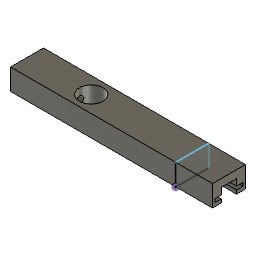
ペン抑え (Autodesk Fusion 360 design; units mm, degrees)
Autodesk Fusion 360 part; units mm, degrees
note: some values were not read from the file. Set by a fixed rule: which sketch regions a step uses.
sketch "スケッチ3" plane through (0, 0, 0) normal (0, 0, 1) x (1, 0, 0)
  line L0 (0, 0) -> (45, 0)
  line L1 (45, 0) -> (45, 9)
  line L2 (45, 9) -> (0, 9)
  line L3 (0, 9) -> (0, 0)
  dimension "d4" = 45
  dimension "d5" = 9
  constraint horizontal L0
  constraint vertical L1
  constraint horizontal L2
  constraint vertical L3
  constraint coincident L0.start L3.end
  measures "d4" distance of L0.start L0.end
  measures "d5" distance of L0.start L2.end
extrude "押し出し2" add sketch "スケッチ3" along normal blind 5.8
sketch "スケッチ4" plane through (0, 0, 0) normal (1, 0, 0) x (0, 1, 0)
sketch "スケッチ5" plane through (45, 0, 0) normal (1, 0, 0) x (0, 1, 0)
  line L0 (0, 0) -> (9, 0)
  line L1 (9, 0) -> (9, 5.8)
  line L2 (9, 5.8) -> (0, 5.8)
  line L3 (0, 5.8) -> (0, 0)
  line L4 (0, 0) -> (0.85, 0)
  line L5 (0.85, 0) -> (0.85, 5.8)
  line L6 (0.85, 5.8) -> (0, 5.8)
  line L7 (0, 5.8) -> (0, 0)
  line L8 (9, 0) -> (8.15, 0)
  line L9 (8.15, 0) -> (8.15, 5.7622)
  line L10 (8.15, 5.7622) -> (9, 5.7622)
  line L11 (9, 5.7622) -> (9, 0)
  line L12 (0.85, 0) -> (8.15, 0)
  line L13 (8.15, 0) -> (8.15, 1)
  line L14 (8.15, 1) -> (0.85, 1)
  line L15 (0.85, 1) -> (0.85, 0)
  line L16 (0.85, 5.8) -> (8.1927, 5.8)
  line L17 (8.1927, 5.8) -> (8.1927, 1.8)
  line L18 (8.1927, 1.8) -> (0.85, 1.8)
  line L19 (0.85, 1.8) -> (0.85, 5.8)
  line L20 (4.5, 1) -> (6.55, 1)
  line L21 (6.55, 1) -> (6.55, 0)
  line L22 (6.55, 0) -> (4.5, 0)
  line L23 (4.5, 0) -> (4.5, 1)
  line L24 (4.5, 0) -> (2.45, 0)
  line L25 (2.45, 0) -> (2.45, 1)
  line L26 (2.45, 1) -> (4.5, 1)
  line L27 (4.5, 1) -> (4.5, 0)
  dimension "d8" = 0.85
  dimension "d9" = 0.85
  dimension "d10" = 1
  dimension "d11" = 4
  dimension "d12" = 2.05
  dimension "d13" = 2.05
  constraint horizontal L4
  constraint vertical L5
  constraint horizontal L6
  constraint vertical L7
  constraint coincident L0.start L3.end
  constraint horizontal L8
  constraint vertical L9
  constraint horizontal L10
  constraint vertical L11
  constraint coincident L0.end L1.start
  constraint horizontal L12
  constraint vertical L13
  constraint horizontal L14
  constraint vertical L15
  constraint horizontal L16
  constraint vertical L17
  constraint horizontal L18
  constraint vertical L19
  constraint horizontal L20
  constraint vertical L21
  constraint horizontal L22
  constraint vertical L23
  constraint midpoint L14 L20.start
  constraint horizontal L24
  constraint vertical L25
  constraint horizontal L26
  constraint vertical L27
  measures "d8" distance of L0.start L4.end
  measures "d9" distance of L0.end L8.end
  measures "d10" distance of L4.end L14.end
  measures "d11" distance of L5.end L18.end
  measures "d12" distance of L20.start L20.end
  measures "d13" distance of L22.end L24.end
sketch "スケッチ6" plane through (0, 0, 5.8) normal (0, 0, 1) x (-1, 0, 0)
  line L0 (0, -9) -> (0, 0)
  line L1 (0, 0) -> (-45, 0)
  line L2 (-45, 0) -> (-45, -9)
  line L3 (-45, -9) -> (0, -9)
  line L4 (-45, -9) -> (-17.5, -9)
  line L5 (-17.5, -9) -> (-17.5, -4.5)
  line L6 (-17.5, -4.5) -> (-45, -4.5)
  line L7 (-45, -4.5) -> (-45, -9)
  circle A0 centre (-17.5, -4.5) radius 3.2
  dimension "d16" = 27.5
  dimension "d17" = 4.5
  dimension "d18" = 6.4
  constraint horizontal L4
  constraint vertical L5
  constraint horizontal L6
  constraint vertical L7
  constraint coincident L2.end L3.start
  constraint coincident L5.end L6.start
  measures "d16" distance of L2.end L4.end
  measures "d17" distance of L2.end L6.end
  measures "d18" diameter of A0
extrude "押し出し4" cut sketch "スケッチ6" against normal blind 9 contours L5 L6 A0 | L5 L6 A0
sketch "スケッチ7" plane through (0, 0, 0) normal (-1, 0, 0) x (0, -1, 0)
  line L0 (-9, 0) -> (0, 0)
  line L1 (0, 0) -> (0, 5.8)
  line L2 (0, 5.8) -> (-9, 5.8)
  line L3 (-9, 5.8) -> (-9, 0)
  line L4 (-9, 0) -> (0, 5.8)
  line L5 (-9, 5.8) -> (0, 0)
  circle A0 centre (-4.5, 2.9) radius 1
  dimension "d21" = 2
  constraint coincident L0.start L3.end
  constraint coincident L1.end L2.start
  constraint coincident L2.end L3.start
  constraint coincident L0.end L1.start
  constraint midpoint L4 A0.centre
  measures "d21" diameter of A0
extrude "押し出し5" cut sketch "スケッチ7" against normal blind 15 contours L4 L5 A0 | L4 L5 A0 | L4 L5 A0 | L4 L5 A0
sketch "スケッチ8" plane through (0, 0, 0) normal (-1, 0, 0) x (0, -1, 0)
  circle A0 centre (-4.5, 2.9) radius 1
  line L0 (-9, 0) -> (0, 0)
  line L1 (0, 0) -> (0, 5.8)
  line L2 (0, 5.8) -> (-9, 5.8)
  line L3 (-9, 5.8) -> (-9, 0)
  circle A1 centre (-4.5, 2.9) radius 1.55
  dimension "d24" = 3.1
  constraint concentric A0 A1
  measures "d24" diameter of A1
extrude "押し出し6" cut sketch "スケッチ8" against normal blind 4 contours A1
sketch "スケッチ9" plane through (45, 0, 0) normal (1, 0, 0) x (0, 1, 0)
  line L0 (9, 0) -> (9, 5.8)
  line L1 (9, 5.8) -> (0, 5.8)
  line L2 (0, 5.8) -> (0, 0)
  line L3 (0, 0) -> (9, 0)
sketch "スケッチ10" plane through (45, 0, 0) normal (1, 0, 0) x (0, 1, 0)
  line L0 (0, 0) -> (9, 0)
  line L1 (9, 0) -> (9, 5.8)
  line L2 (9, 5.8) -> (0, 5.8)
  line L3 (0, 5.8) -> (0, 0)
  constraint horizontal L0
  constraint vertical L1
  constraint horizontal L2
  constraint vertical L3
  constraint coincident L0.start L3.end
extrude "押し出し7" add sketch "スケッチ9" along normal blind 10
sketch "スケッチ11" plane through (55, 0, 0) normal (1, 0, 0) x (0, 1, 0)
  line L0 (0, 0) -> (9, 0)
  line L1 (9, 0) -> (9, 5.8)
  line L2 (9, 5.8) -> (0, 5.8)
  line L3 (0, 5.8) -> (0, 0)
  line L4 (0, 0) -> (4.5, 0)
  line L5 (4.5, 0) -> (6.55, 0)
  line L6 (6.55, 0) -> (6.55, 1)
  line L7 (6.55, 1) -> (4.5, 1)
  line L8 (4.5, 1) -> (4.5, 0)
  line L9 (4.5, 0) -> (2.45, 0)
  line L10 (2.45, 0) -> (2.45, 1)
  line L11 (2.45, 1) -> (4.5, 1)
  line L12 (4.5, 1) -> (4.5, 0)
  line L13 (9, 0) -> (8.3, 0)
  line L14 (8.3, 0) -> (8.3, 5.8)
  line L15 (8.3, 5.8) -> (9, 5.8)
  line L16 (9, 5.8) -> (9, 0)
  line L17 (0, 0) -> (0.7, 0)
  line L18 (0.7, 0) -> (0.7, 5.8)
  line L19 (0.7, 5.8) -> (0, 5.8)
  line L20 (0, 5.8) -> (0, 0)
  line L21 (0.7, 1) -> (8.3, 1)
  line L22 (8.3, 1) -> (8.3, 1.9)
  line L23 (8.3, 1.9) -> (0.7, 1.9)
  line L24 (0.7, 1.9) -> (0.7, 1)
  line L25 (4.5, 1.9) -> (6.55, 1.9)
  line L26 (6.55, 1.9) -> (6.55, 4.9)
  line L27 (6.55, 4.9) -> (4.5, 4.9)
  line L28 (4.5, 4.9) -> (4.5, 1.9)
  line L29 (4.5, 1.9) -> (2.45, 1.9)
  line L30 (2.45, 1.9) -> (2.45, 4.9)
  line L31 (2.45, 4.9) -> (4.5, 4.9)
  line L32 (4.5, 4.9) -> (4.5, 1.9)
  dimension "d29" = 4.5
  dimension "d30" = 2.05
  dimension "d31" = 1
  dimension "d32" = 0.9
  dimension "d33" = 2.05
  dimension "d34" = 3
  dimension "d35" = 2.05
  constraint coincident L0.start L3.end
  constraint perpendicular L3 L4
  constraint horizontal L5
  constraint vertical L6
  constraint horizontal L7
  constraint vertical L8
  constraint horizontal L9
  constraint vertical L10
  constraint horizontal L11
  constraint vertical L12
  constraint horizontal L13
  constraint vertical L14
  constraint horizontal L15
  constraint vertical L16
  constraint coincident L2 L14.end
  constraint coincident L0.end L1.start
  constraint horizontal L17
  constraint vertical L18
  constraint horizontal L19
  constraint vertical L20
  constraint coincident L2 L18.end
  constraint horizontal L21
  constraint vertical L22
  constraint horizontal L23
  constraint vertical L24
  constraint coincident L18 L21.start
  constraint horizontal L25
  constraint vertical L26
  constraint horizontal L27
  constraint vertical L28
  constraint midpoint L23 L25.start
  constraint horizontal L29
  constraint vertical L30
  constraint horizontal L31
  constraint vertical L32
  measures "d29" distance of L0.start L4.end
  measures "d30" distance of L4.end L5.end
  measures "d31" distance of L4.end L7.end
  measures "d32" distance of L21.start L23.end
  measures "d33" distance of L25.start L25.end
  measures "d34" distance of L25.start L27.end
  measures "d35" distance of L25.start L29.end
extrude "押し出し8" cut sketch "スケッチ11" against normal blind 28 contours L0 L4 L8 L9 L10 L11 L12 L21 | L7 L11 L14 L18 L21 L22 L23 L24 L25 L29 | L0 L5 L6 L7 L8 L12 L21 | L23 L28 L29 L30 L31 L32 | L23 L25 L26 L27 L28 L32
sketch "スケッチ12" plane through (0, 0, 4.9) normal (0, 0, -1) x (1, 0, 0)
  line L0 (55, -6.55) -> (55, -2.45)
  line L1 (55, -2.45) -> (27, -2.45)
  line L2 (27, -2.45) -> (27, -6.55)
  line L3 (27, -6.55) -> (55, -6.55)
  line L4 (55, -6.55) -> (27, -6.55)
  line L5 (27, -6.55) -> (27, -2.45)
  line L6 (27, -2.45) -> (55, -2.45)
  line L7 (55, -2.45) -> (55, -6.55)
  constraint horizontal L4
  constraint vertical L5
  constraint horizontal L6
  constraint vertical L7
  constraint coincident L1.end L2.start
  constraint coincident L0.start L3.end
extrude "押し出し9" add sketch "スケッチ12" along normal blind 1.2
